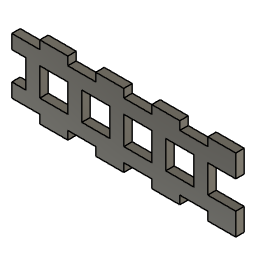
DiceHolder_FrontWall_V2 v2 (Autodesk Fusion 360 design; units mm, degrees)
Autodesk Fusion 360 part; units mm, degrees
note: some values were not read from the file. Set by a fixed rule: which face or edge a step refers to.
sketch "Sketch1" plane through (0, 0, 0) normal (0, 1, 0) x (1, 0, 0)
  line L0 (50, -10) -> (-50, -10)
  line L1 (-50, -10) -> (-50, 10)
  line L2 (-50, 10) -> (50, 10)
  line L3 (50, 10) -> (50, -10)
  line L4 (50, -10) -> (-50, 10) construction
  line L5 (-50, -10) -> (50, 10) construction
  dimension "d1" = 100
  dimension "d2" = 20
  constraint horizontal L0
  constraint perpendicular L0 L1
  constraint parallel L0 L2
  constraint parallel L1 L3
  constraint coincident L4 origin
  constraint coincident L5 origin
  measures "d1" distance of L1.end L2.end
  measures "d2" distance of L0.end L1.end
extrude "Extrude1" add sketch "Sketch1" along normal blind 3
sketch "Sketch2" plane through (0, 3, 0) normal (0, 1, 0) x (-1, 0, 0)
  line L0 (-50, -10) -> (50, -10)
  line L1 (50, -10) -> (50, 10)
  line L2 (50, 10) -> (-50, 10)
  line L3 (-50, 10) -> (-50, -10)
  line L4 (-50, -10) -> (-40, -10) construction
  line L5 (-40, -10) -> (-40, -7) construction
  line L6 (-40, -7) -> (-50, -7) construction
  line L7 (-50, -7) -> (-50, -10) construction
  line L8 (-40, -10) -> (-30, -10)
  line L9 (-30, -10) -> (-30, -7)
  line L10 (-30, -7) -> (-40, -7)
  line L11 (-40, -7) -> (-40, -10)
  constraint horizontal L4
  constraint vertical L5
  constraint horizontal L6
  constraint vertical L7
  constraint coincident L0.start L3.end
  constraint horizontal L8
  constraint vertical L9
  constraint horizontal L10
  constraint vertical L11
extrude "Extrude2" cut sketch "Sketch2" against normal blind 6 contours L0 L8 L9 L10 L11
pattern_linear "R-Pattern1" count 5 spacing 20 along (-1, 0, 0) count 2 spacing 17 along (0, 0, 1) of "Extrude2"
extrude "Extrude3" add 5 faces at (43.3333, 2, 10) (26.6667, 1, 10) (6.6667, 1, 10) (-13.3333, 1, 10) (-33.3333, 1, 10) along direction (0, 0, 1) blind 3
extrude "Extrude4" add 5 faces at (36.6667, 2, 7) (16.6667, 2, 7) (-3.3333, 2, 7) (-23.3333, 2, 7) (-46.6667, 1, 7) along direction (0, 0, 1) blind 3
extrude "Extrude5" add 5 faces at (43.3333, 1, -10) (23.3333, 1, -10) (-36.6667, 1, -10) (-16.6667, 1, -10) (3.3333, 1, -10) along direction (0, 0, -1) blind 3
extrude "Extrude6" add 5 faces at (33.3333, 2, -7) (-26.6667, 2, -7) (-43.3333, 1, -7) (13.3333, 2, -7) (-6.6667, 2, -7) along direction (0, 0, -1) blind 3
sketch "Sketch3" plane through (0, 3, 0) normal (0, 1, 0) x (-1, 0, 0)
  line L0 (40, 10) -> (40, 13)
  line L1 (40, 13) -> (30, 13)
  line L2 (30, 13) -> (30, 10)
  line L3 (30, 10) -> (20, 10)
  line L4 (20, 10) -> (20, 13)
  line L5 (20, 13) -> (10, 13)
  line L6 (10, 13) -> (10, 10)
  line L7 (10, 10) -> (0, 10)
  line L8 (0, 10) -> (0, 13)
  line L9 (0, 13) -> (-10, 13)
  line L10 (-10, 13) -> (-10, 10)
  line L11 (-10, 10) -> (-20, 10)
  line L12 (-20, 10) -> (-20, 13)
  line L13 (-20, 13) -> (-30, 13)
  line L14 (-30, 13) -> (-30, 10)
  line L15 (-30, 10) -> (-40, 10)
  line L16 (-40, 10) -> (-40, 13)
  line L17 (-40, 13) -> (-50, 13)
  line L18 (-50, 13) -> (-50, -13)
  line L19 (-50, -13) -> (-40, -13)
  line L20 (-40, -13) -> (-40, -10)
  line L21 (-40, -10) -> (-30, -10)
  line L22 (-30, -10) -> (-30, -13)
  line L23 (-30, -13) -> (-20, -13)
  line L24 (-20, -13) -> (-20, -10)
  line L25 (-20, -10) -> (-10, -10)
  line L26 (-10, -10) -> (-10, -13)
  line L27 (-10, -13) -> (0, -13)
  line L28 (0, -13) -> (0, -10)
  line L29 (0, -10) -> (10, -10)
  line L30 (10, -10) -> (10, -13)
  line L31 (10, -13) -> (20, -13)
  line L32 (20, -13) -> (20, -10)
  line L33 (20, -10) -> (30, -10)
  line L34 (30, -10) -> (30, -13)
  line L35 (30, -13) -> (40, -13)
  line L36 (40, -13) -> (40, -10)
  line L37 (40, -10) -> (50, -10)
  line L38 (50, -10) -> (50, 10)
  line L39 (50, 10) -> (40, 10)
  line L40 (-40, -5) -> (-50, -5)
  line L41 (-50, -5) -> (-50, 5)
  line L42 (-50, 5) -> (-40, 5)
  line L43 (-40, 5) -> (-40, -5)
  line L44 (-40, -5) -> (-50, 5) construction
  line L45 (-50, -5) -> (-40, 5) construction
  line L46 (-25, -5) -> (-35, -5)
  line L47 (-35, -5) -> (-35, 5)
  line L48 (-35, 5) -> (-25, 5)
  line L49 (-25, 5) -> (-25, -5)
  line L50 (-25, -5) -> (-35, 5) construction
  line L51 (-35, -5) -> (-25, 5) construction
  line L52 (-10, -5) -> (-20, -5)
  line L53 (-20, -5) -> (-20, 5)
  line L54 (-20, 5) -> (-10, 5)
  line L55 (-10, 5) -> (-10, -5)
  line L56 (-10, -5) -> (-20, 5) construction
  line L57 (-20, -5) -> (-10, 5) construction
  line L58 (5, -5) -> (-5, -5)
  line L59 (-5, -5) -> (-5, 5)
  line L60 (-5, 5) -> (5, 5)
  line L61 (5, 5) -> (5, -5)
  line L62 (5, -5) -> (-5, 5) construction
  line L63 (-5, -5) -> (5, 5) construction
  line L64 (20, -5) -> (10, -5)
  line L65 (10, -5) -> (10, 5)
  line L66 (10, 5) -> (20, 5)
  line L67 (20, 5) -> (20, -5)
  line L68 (20, -5) -> (10, 5) construction
  line L69 (10, -5) -> (20, 5) construction
  line L70 (35, -5) -> (25, -5)
  line L71 (25, -5) -> (25, 5)
  line L72 (25, 5) -> (35, 5)
  line L73 (35, 5) -> (35, -5)
  line L74 (35, -5) -> (25, 5) construction
  line L75 (25, -5) -> (35, 5) construction
  line L76 (50, -5) -> (40, -5)
  line L77 (40, -5) -> (40, 5)
  line L78 (40, 5) -> (50, 5)
  line L79 (50, 5) -> (50, -5)
  line L80 (50, -5) -> (40, 5) construction
  line L81 (40, -5) -> (50, 5) construction
  point P0 (-45, 0)
  point P1 (-30, 0)
  point P2 (-15, 0)
  point P3 (15, 0)
  point P4 (30, 0)
  point P5 (45, 0)
  constraint horizontal L40
  constraint perpendicular L40 L41
  constraint parallel L40 L42
  constraint parallel L41 L43
  constraint coincident L44 P0
  constraint coincident L45 P0
  constraint horizontal L46
  constraint perpendicular L46 L47
  constraint parallel L46 L48
  constraint parallel L47 L49
  constraint coincident L50 P1
  constraint coincident L51 P1
  constraint horizontal L52
  constraint perpendicular L52 L53
  constraint parallel L52 L54
  constraint parallel L53 L55
  constraint coincident L56 P2
  constraint coincident L57 P2
  constraint horizontal L58
  constraint perpendicular L58 L59
  constraint parallel L58 L60
  constraint parallel L59 L61
  constraint coincident L62 origin
  constraint coincident L63 origin
  constraint horizontal L64
  constraint perpendicular L64 L65
  constraint parallel L64 L66
  constraint parallel L65 L67
  constraint coincident L68 P3
  constraint coincident L69 P3
  constraint horizontal L70
  constraint perpendicular L70 L71
  constraint parallel L70 L72
  constraint parallel L71 L73
  constraint coincident L74 P4
  constraint coincident L75 P4
  constraint horizontal L76
  constraint perpendicular L76 L77
  constraint parallel L76 L78
  constraint parallel L77 L79
  constraint coincident L80 P5
  constraint coincident L81 P5
  constraint coincident L38 L76.start
extrude "Extrude7" cut sketch "Sketch3" against normal blind 20 contours L38 L76 L77 L78 L79 | L46 L47 L48 L49 | L52 L53 L54 L55 | L58 L59 L60 L61 | L64 L65 L66 L67 | L70 L71 L72 L73
sketch "Sketch4" plane through (0, 3, 0) normal (0, 1, 0) x (-1, 0, 0)
  line L0 (40, 5) -> (50, 5)
  line L1 (50, 5) -> (50, 10)
  line L2 (50, 10) -> (40, 10)
  line L3 (40, 10) -> (40, 13)
  line L4 (40, 13) -> (30, 13)
  line L5 (30, 13) -> (30, 10)
  line L6 (30, 10) -> (20, 10)
  line L7 (20, 10) -> (20, 13)
  line L8 (20, 13) -> (10, 13)
  line L9 (10, 13) -> (10, 10)
  line L10 (10, 10) -> (0, 10)
  line L11 (0, 10) -> (0, 13)
  line L12 (0, 13) -> (-10, 13)
  line L13 (-10, 13) -> (-10, 10)
  line L14 (-10, 10) -> (-20, 10)
  line L15 (-20, 10) -> (-20, 13)
  line L16 (-20, 13) -> (-30, 13)
  line L17 (-30, 13) -> (-30, 10)
  line L18 (-30, 10) -> (-40, 10)
  line L19 (-40, 10) -> (-40, 13)
  line L20 (-40, 13) -> (-50, 13)
  line L21 (-50, 13) -> (-50, -13)
  line L22 (-50, -13) -> (-40, -13)
  line L23 (-40, -13) -> (-40, -10)
  line L24 (-40, -10) -> (-30, -10)
  line L25 (-30, -10) -> (-30, -13)
  line L26 (-30, -13) -> (-20, -13)
  line L27 (-20, -13) -> (-20, -10)
  line L28 (-20, -10) -> (-10, -10)
  line L29 (-10, -10) -> (-10, -13)
  line L30 (-10, -13) -> (0, -13)
  line L31 (0, -13) -> (0, -10)
  line L32 (0, -10) -> (10, -10)
  line L33 (10, -10) -> (10, -13)
  line L34 (10, -13) -> (20, -13)
  line L35 (20, -13) -> (20, -10)
  line L36 (20, -10) -> (30, -10)
  line L37 (30, -10) -> (30, -13)
  line L38 (30, -13) -> (40, -13)
  line L39 (40, -13) -> (40, -10)
  line L40 (40, -10) -> (50, -10)
  line L41 (50, -10) -> (50, -5)
  line L42 (50, -5) -> (40, -5)
  line L43 (40, -5) -> (40, 5)
  line L44 (10, -5) -> (10, 5)
  line L45 (10, 5) -> (20, 5)
  line L46 (20, 5) -> (20, -5)
  line L47 (20, -5) -> (10, -5)
  line L48 (-35, -5) -> (-35, 5)
  line L49 (-35, 5) -> (-25, 5)
  line L50 (-25, 5) -> (-25, -5)
  line L51 (-25, -5) -> (-35, -5)
  line L52 (25, -5) -> (25, 5)
  line L53 (25, 5) -> (35, 5)
  line L54 (35, 5) -> (35, -5)
  line L55 (35, -5) -> (25, -5)
  line L56 (-5, -5) -> (-5, 5)
  line L57 (-5, 5) -> (5, 5)
  line L58 (5, 5) -> (5, -5)
  line L59 (5, -5) -> (-5, -5)
  line L60 (-20, -5) -> (-20, 5)
  line L61 (-20, 5) -> (-10, 5)
  line L62 (-10, 5) -> (-10, -5)
  line L63 (-10, -5) -> (-20, -5)
  line L64 (-40, -5) -> (-50, -5)
  line L65 (-50, -5) -> (-50, 5)
  line L66 (-50, 5) -> (-40, 5)
  line L67 (-40, 5) -> (-40, -5)
  line L68 (-40, -5) -> (-50, 5) construction
  line L69 (-50, -5) -> (-40, 5) construction
  point P0 (-45, 0)
  constraint horizontal L64
  constraint perpendicular L64 L65
  constraint parallel L64 L66
  constraint parallel L65 L67
  constraint coincident L68 P0
  constraint coincident L69 P0
extrude "Extrude8" cut sketch "Sketch4" against normal blind 25 contours L21 L64 L65 L66 L67
sketch "Sketch5" plane through (0, 0, 0) normal (0, -1, 0) x (1, 0, 0)
  line L0 (-10, 5) -> (-10, -5)
  line L1 (-10, -5) -> (-20, -5)
  line L2 (-20, -5) -> (-20, 5)
  line L3 (-20, 5) -> (-10, 5)
  line L4 (35, 5) -> (35, -5)
  line L5 (35, -5) -> (25, -5)
  line L6 (25, -5) -> (25, 5)
  line L7 (25, 5) -> (35, 5)
  line L8 (-25, 5) -> (-25, -5)
  line L9 (-25, -5) -> (-35, -5)
  line L10 (-35, -5) -> (-35, 5)
  line L11 (-35, 5) -> (-25, 5)
  line L12 (5, 5) -> (5, -5)
  line L13 (5, -5) -> (-5, -5)
  line L14 (-5, -5) -> (-5, 5)
  line L15 (-5, 5) -> (5, 5)
  line L16 (20, 5) -> (20, -5)
  line L17 (20, -5) -> (10, -5)
  line L18 (10, -5) -> (10, 5)
  line L19 (10, 5) -> (20, 5)
  line L20 (50, -5) -> (40, -5)
  line L21 (40, -5) -> (40, 5)
  line L22 (40, 5) -> (50, 5)
  line L23 (50, 5) -> (50, 13)
  line L24 (50, 13) -> (40, 13)
  line L25 (40, 13) -> (40, 10)
  line L26 (40, 10) -> (30, 10)
  line L27 (30, 10) -> (30, 13)
  line L28 (30, 13) -> (20, 13)
  line L29 (20, 13) -> (20, 10)
  line L30 (20, 10) -> (10, 10)
  line L31 (10, 10) -> (10, 13)
  line L32 (10, 13) -> (0, 13)
  line L33 (0, 13) -> (0, 10)
  line L34 (0, 10) -> (-10, 10)
  line L35 (-10, 10) -> (-10, 13)
  line L36 (-10, 13) -> (-20, 13)
  line L37 (-20, 13) -> (-20, 10)
  line L38 (-20, 10) -> (-30, 10)
  line L39 (-30, 10) -> (-30, 13)
  line L40 (-30, 13) -> (-40, 13)
  line L41 (-40, 13) -> (-40, 10)
  line L42 (-40, 10) -> (-50, 10)
  line L43 (-50, 10) -> (-50, 5)
  line L44 (-50, 5) -> (-40, 5)
  line L45 (-40, 5) -> (-40, -5)
  line L46 (-40, -5) -> (-50, -5)
  line L47 (-50, -5) -> (-50, -10)
  line L48 (-50, -10) -> (-40, -10)
  line L49 (-40, -10) -> (-40, -13)
  line L50 (-40, -13) -> (-30, -13)
  line L51 (-30, -13) -> (-30, -10)
  line L52 (-30, -10) -> (-20, -10)
  line L53 (-20, -10) -> (-20, -13)
  line L54 (-20, -13) -> (-10, -13)
  line L55 (-10, -13) -> (-10, -10)
  line L56 (-10, -10) -> (0, -10)
  line L57 (0, -10) -> (0, -13)
  line L58 (0, -13) -> (10, -13)
  line L59 (10, -13) -> (10, -10)
  line L60 (10, -10) -> (20, -10)
  line L61 (20, -10) -> (20, -13)
  line L62 (20, -13) -> (30, -13)
  line L63 (30, -13) -> (30, -10)
  line L64 (30, -10) -> (40, -10)
  line L65 (40, -10) -> (40, -13)
  line L66 (40, -13) -> (50, -13)
  line L67 (50, -13) -> (50, -5)
  line L68 (-30, 29) -> (-56, 29)
  line L69 (-56, 29) -> (-56, -29)
  line L70 (-56, -29) -> (-30, -29)
  line L71 (-30, -29) -> (-30, 29)
  line L72 (-30, 29) -> (-56, -29) construction
  line L73 (-56, 29) -> (-30, -29) construction
  point P0 (-43, 0)
  constraint horizontal L68
  constraint perpendicular L68 L69
  constraint parallel L68 L70
  constraint parallel L69 L71
  constraint coincident L72 P0
  constraint coincident L73 P0
extrude "Extrude9" cut sketch "Sketch5" against normal blind 66 contours L9 L10 L11 L39 L40 L41 L42 L43 L44 L45 L46 L47 L48 L49 L50 L51 L71
